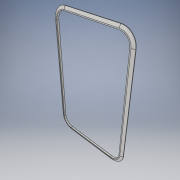
# Autodesk Inventor part: FrontPanelBezel
Saved by Autodesk Inventor 2019 (Build 230136000, 136)
## iProperties
Created: 2025-01-22
Part Number: FrontPanelBezel
Material: Générique
Document SubType Name: Modeling
Designer: Maxime
Density: 1 g/cm^3
Appearance: Par défaut
Author: Maxime
Autodesk Inventor part; units mm, degrees
ref_plane "YZ Plane" through (0, 0, 0) normal (1, 0, 0) x (0, 1, 0)
ref_plane "XZ Plane" through (0, 0, 0) normal (0, 1, 0) x (-1, 0, 0)
ref_plane "XY Plane" through (0, 0, 0) normal (0, 0, 1) x (1, 0, 0)
sketch "Esquisse1" plane through (0, 0, 0) normal (0, 0, 1) x (1, 0, 0)
  line L0 (33.2, -53.2) -> (-33.2, -53.2)
  line L1 (-33.2, -53.2) -> (-33.2, 53.2)
  line L2 (-33.2, 53.2) -> (33.2, 53.2)
  line L3 (33.2, 53.2) -> (33.2, -53.2)
  line L4 (33.2, -53.2) -> (-33.2, 53.2) construction
  line L5 (-33.2, -53.2) -> (33.2, 53.2) construction
  line L6 (30.2, 50.2) -> (-30.2, 50.2)
  line L7 (-30.2, 50.2) -> (-30.2, -50.2)
  line L8 (-30.2, -50.2) -> (30.2, -50.2)
  line L9 (30.2, -50.2) -> (30.2, 50.2)
  point P0 (0, 0)
  dimension "d0" = 66.4
  dimension "d1" = 106.4
  dimension "d2" = 3
  constraints: 20 end point, 4 parallel, 2 midpoint, 2 perpendicular, 1 horizontal, 3 other
  measures "d0" distance of L1.end L2.end
  measures "d1" distance of L0.end L1.end
  measures "d2" distance between parallel lines of L2 L6
extrude "Extrusion1" add sketch "Esquisse1" along normal blind 1.6
fillet "Congé1" radius 11 4 edges at (-33.2, 53.2, 0.8) (33.2, 53.2, 0.8) (33.2, -53.2, 0.8) (-33.2, -53.2, 0.8)
fillet "Congé1" radius 8 4 edges at (30.2, -50.2, 0.8) (-30.2, -50.2, 0.8) (-30.2, 50.2, 0.8) (30.2, 50.2, 0.8)
chamfer "Chanfrein1" distance 2.2 distance2 1.15 8 edges at (-33.2, 0, 1.6) (-29.9782, -49.9782, 1.6) (0, -53.2, 1.6) (29.9782, -49.9782, 1.6) (33.2, 0, 1.6) (29.9782, 49.9782, 1.6) (0, 53.2, 1.6) (-29.9782, 49.9782, 1.6) measured on face at (-31.2, 14.0667, 1.6)
